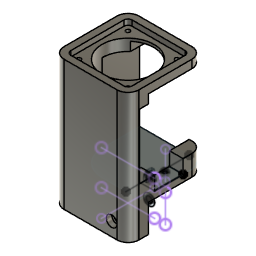
motor-profile connector R (Autodesk Fusion 360 design; units mm, degrees)
Autodesk Fusion 360 part; units mm, degrees
sketch "Sketch1" plane through (0, 0, 0) normal (0, 0, 1) x (1, 0, 0)
  circle A0 centre (0, 0) radius 19
  line L0 (19.5, -22.5) -> (-19.5, -22.5)
  line L1 (-22.5, -19.5) -> (-22.5, 19.5)
  line L2 (-19.5, 22.5) -> (19.5, 22.5)
  line L3 (22.5, 19.5) -> (22.5, -19.5)
  line L4 (22.5, -22.5) -> (-22.5, 22.5) construction
  line L5 (-22.5, -22.5) -> (22.5, 22.5) construction
  line L6 (-2.5, 36.7573) -> (-2.5, -35)
  line L7 (-2.5, -35) -> (-2.5, 36.7573)
  line L8 (-35.201, -2.5) -> (35, -2.5)
  line L9 (35, -2.5) -> (-35.201, -2.5)
  line L10 (7.5, 7.5) -> (62.5, 7.5)
  line L11 (62.5, 7.5) -> (62.5, -12.5)
  line L12 (62.5, -12.5) -> (7.5, -12.5)
  line L13 (7.5, -12.5) -> (7.5, 7.5)
  line L14 (7.5, 7.5) -> (62.5, -12.5) construction
  line L15 (62.5, 7.5) -> (7.5, -12.5) construction
  line L16 (7.5, 7.5) -> (-12.5, 7.5)
  line L17 (-12.5, 7.5) -> (-12.5, 66.0146)
  line L18 (-12.5, 66.0146) -> (7.5, 66.0146)
  line L19 (7.5, 66.0146) -> (7.5, 7.5)
  line L20 (7.5, 7.5) -> (-12.5, 66.0146) construction
  line L21 (-12.5, 7.5) -> (7.5, 66.0146) construction
  circle A1 centre (-18, 18) radius 1.5
  circle A2 centre (18, 18) radius 1.5
  circle A3 centre (-18, -18) radius 1.5
  circle A4 centre (18, -18) radius 1.5
  line L22 (-12.5, 7.5) -> (-12.5, -12.5)
  line L23 (-12.5, -12.5) -> (7.5, -12.5)
  arc A5 (-19.5, 22.5) -> (-22.5, 19.5) centre (-19.5, 19.5) ccw
  arc A6 (-22.5, -19.5) -> (-19.5, -22.5) centre (-19.5, -19.5) ccw
  arc A7 (19.5, -22.5) -> (22.5, -19.5) centre (19.5, -19.5) ccw
  arc A8 (22.5, 19.5) -> (19.5, 22.5) centre (19.5, 19.5) ccw
  arc A9 (-27.5, -19.5) -> (-19.5, -27.5) centre (-19.5, -19.5) ccw
  line L24 (19.5, -27.5) -> (-19.5, -27.5)
  arc A10 (19.5, -27.5) -> (27.5, -19.5) centre (19.5, -19.5) ccw
  line L25 (27.5, 19.5) -> (27.5, -19.5)
  arc A11 (27.5, 19.5) -> (19.5, 27.5) centre (19.5, 19.5) ccw
  line L26 (-19.5, 27.5) -> (19.5, 27.5)
  arc A12 (-19.5, 27.5) -> (-27.5, 19.5) centre (-19.5, 19.5) ccw
  line L27 (-27.5, -19.5) -> (-27.5, 19.5)
  line L28 (-19, 0) -> (-19, 27.5)
  line L29 (0, -19) -> (27.5, -19)
  circle A13 centre (-7, 0) radius 6.5
  point P0 (35, -2.5)
  point P1 (-2.5, 36.7573)
  dimension "d1" = 38
  dimension "d2" = 45
  dimension "d3" = 45
  dimension "d4" = 2.5
  dimension "d5" = 2.5
  dimension "d6" = 20
  dimension "d7" = 4.5
  dimension "d8" = 4.5
  dimension "d9" = 4.5
  dimension "d10" = 4.5
  dimension "d11" = 3
  dimension "d12" = 3
  dimension "d13" = 3
  dimension "d14" = 3
  dimension "d17" = 3
  dimension "d26" = -5
  dimension "d33" = 7
  dimension "d34" = 13
  constraint coincident A0.centre origin
  constraint horizontal L0
  constraint perpendicular L0 L1
  constraint parallel L0 L2
  constraint parallel L1 L3
  constraint coincident L4 A0.centre
  constraint coincident L5 A0.centre
  constraint perpendicular L0 L6
  constraint perpendicular L1 L8
  constraint horizontal L10
  constraint perpendicular L10 L11
  constraint parallel L10 L12
  constraint parallel L11 L13
  constraint coincident L14 P0
  constraint coincident L15 P0
  constraint coincident L5 L10.start
  constraint coincident P0 L8.end
  constraint horizontal L16
  constraint perpendicular L16 L17
  constraint parallel L16 L18
  constraint parallel L17 L19
  constraint coincident L20 P1
  constraint coincident L21 P1
  constraint coincident P1 L6.start
  constraint coincident L4 A1.centre
  constraint coincident L5 A2.centre
  constraint coincident L5 A3.centre
  constraint coincident L4 A4.centre
  constraint coincident L5 L22.end
  constraint perpendicular L16 L22
  constraint coincident L4.end L2
  constraint coincident L4.end L1
  constraint tangent L2 A5
  constraint tangent L1 A5
  constraint coincident L5.start L1
  constraint coincident L5.start L0
  constraint tangent L1 A6
  constraint tangent L0 A6
  constraint equal A5 A6
  constraint coincident L4.start L0
  constraint coincident L4.start L3
  constraint tangent L0 A7
  constraint tangent L3 A7
  constraint equal A5 A7
  constraint coincident L5.end L2
  constraint coincident L5.end L3
  constraint tangent L2 A8
  constraint tangent L3 A8
  constraint equal A5 A8
  constraint coincident A0 L28.start
  constraint coincident L26 L28.end
  constraint perpendicular L26 L28
  constraint coincident A0 L29.start
  constraint coincident L25 L29.end
  constraint perpendicular L25 L29
  measures "d1" diameter of A0
  measures "d2" distance of L4.end L5.end
  measures "d3" distance of L4.start L5.end
  measures "d4" distance of A0.centre L7
  measures "d5" distance of A0.centre L8
  measures "d6" distance of L17.end L18.end
  measures "d7" distance of L2 A1.centre
  measures "d8" distance of L2 A2.centre
  measures "d9" distance of L0 A3.centre
  measures "d10" distance of L0 A4.centre
  measures "d11" diameter of A1
  measures "d12" diameter of A2
  measures "d13" diameter of A4
  measures "d14" diameter of A3
  measures "d17" radius of A5
  measures "d33" distance of A0.centre A13.centre
  measures "d34" diameter of A13
extrude "Extrude1" add sketch "Sketch1" along normal blind 95.5 contours A0 L3 L12 A4 L29 | A0 L6 L7 L12 L23 | A0 L0 L3 L6 L7 A4 A7 L29 | L3 L12 L25 L29 | A0 L8 L9 L17 L22 A13 | A0 L2 L17 A1 L28 | A0 L0 L1 L6 L7 L8 L9 A6 | A0 L6 L7 L8 L9 L22 L23 A13 | A4 L29 | A4 L29 | L0 L3 L6 L7 A7 L24 A10 L25 L29 | A0 L1 L2 L8 L9 A1 A5 L28 | L2 L17 L26 L28 | L8 L9 L22 A13 | L0 L1 L6 L7 L8 L9 A6 A9 L24 L27 | L8 L9 L22 A13 | A1 L28 | A1 L28 | L1 L2 L8 L9 A5 L26 A12 L27 L28 | A3
extrude "Extrude2" add sketch "Sketch1" along normal blind 6 from surface at 89.5 contours A0 L3 L8 L9 L10 | A0 L2 L3 L10 L19 A8 | A0 L3 L8 L9 L12 | A0 L2 L6 L7 L19 | L3 L8 L9 L10 L25 | L2 L3 L10 L19 A8 L25 A11 L26 | A0 L3 L12 A4 L29 | L3 L8 L9 L12 L25 | A0 L2 L6 L7 L17 | L2 L6 L7 L19 L26 | A0 L0 L3 L6 L7 A4 A7 L29 | L3 L12 L25 L29 | A0 L2 L17 A1 L28 | L2 L6 L7 L17 L26 | A0 L0 L1 L6 L7 L8 L9 A6 | A4 L29 | A4 L29 | L0 L3 L6 L7 A7 L24 A10 L25 L29 | A0 L1 L2 L8 L9 A1 A5 L28 | L2 L17 L26 L28 | L0 L1 L6 L7 L8 L9 A6 A9 L24 L27 | A1 L28 | A1 L28 | L1 L2 L8 L9 A5 L26 A12 L27 L28 | A2 | A3
extrude "Extrude5" cut sketch "Sketch1" along normal blind 4 from surface at 91.5 contours A0 L8 L9 L10 L13 | A0 L3 L8 L9 L10 | A0 L10 L19 | A0 L2 L3 L10 L19 A8 | A0 L3 L8 L9 L12 | A0 L8 L9 L12 L13 | A0 L6 L7 L16 L19 | A0 L2 L6 L7 L19 | L6 L7 L8 L9 L13 L16 A13 | A0 L3 L12 A4 L29 | A0 L6 L7 L12 L23 | L6 L7 L8 L9 L13 L23 A13 | A0 L6 L7 L16 L17 | A0 L2 L6 L7 L17 | L6 L7 L16 L22 A13 | A0 L0 L3 L6 L7 A4 A7 L29 | L6 L7 L8 L9 A13 | L6 L7 L8 L9 A13 | A0 L8 L9 L17 L22 A13 | A0 L2 L17 A1 L28 | L6 L7 L8 L9 L22 A13 | A0 L0 L1 L6 L7 L8 L9 A6 | A0 L6 L7 L8 L9 L22 L23 A13 | A4 L29 | A4 L29 | L6 L7 L22 L23 A13 | L6 L7 L8 L9 L22 A13 | A0 L1 L2 L8 L9 A1 A5 L28 | L8 L9 L22 A13 | L8 L9 L22 A13 | A1 L28 | A1 L28 | A2 | A3
extrude "Extrude3" cut sketch "Sketch1" along normal blind 8 from surface at 83.5 contours A4 L29 | A4 L29 | A1 L28 | A1 L28 | A2 | A3
extrude "Extrude4" cut sketch "Sketch1" along normal through all from surface at 20.5 contours A0 L8 L9 L10 L13 | A0 L10 L19 | A0 L8 L9 L12 L13 | A0 L6 L7 L16 L19 | L6 L7 L8 L9 L13 L16 A13 | A0 L6 L7 L12 L23 | L6 L7 L8 L9 L13 L23 A13 | A0 L6 L7 L16 L17 | L6 L7 L16 L22 A13 | L6 L7 L8 L9 A13 | L6 L7 L8 L9 A13 | A0 L8 L9 L17 L22 A13 | L6 L7 L8 L9 L22 A13 | A0 L6 L7 L8 L9 L22 L23 A13 | L6 L7 L22 L23 A13 | L6 L7 L8 L9 L22 A13 | L8 L9 L22 A13 | L8 L9 L22 A13
extrude "Extrude6" cut sketch "Sketch1" along normal blind 62.5 from surface at 20.5 contours A0 L3 L12 A4 L29 | L3 L12 L25 L29 | A0 L2 L17 A1 L28 | A4 L29 | L2 L17 L26 L28 | A1 L28 picked at (17.9212, -18.1088) picked at (-18.2904, 18.3293)
extrude "Extrude7" add sketch "Sketch1" 1 faces at (-17.5, 11.5, 0) along normal blind 5 from surface at 20.5 contours A0 L8 L9 L10 L13 | A0 L3 L8 L9 L10 | A0 L10 L19 | A0 L2 L3 L10 L19 A8 | A0 L3 L8 L9 L12 | A0 L8 L9 L12 L13 | A0 L6 L7 L16 L19 | A0 L2 L6 L7 L19 | L6 L7 L8 L9 L13 L16 A13 | L3 L8 L9 L10 L25 | L2 L3 L10 L19 A8 L25 A11 L26 | A0 L3 L12 A4 L29 | A0 L6 L7 L12 L23 | L6 L7 L8 L9 L13 L23 A13 | L3 L8 L9 L12 L25 | A0 L6 L7 L16 L17 | A0 L2 L6 L7 L17 | L2 L6 L7 L19 L26 | L6 L7 L16 L22 A13 | L3 L12 L25 L29 | L6 L7 L8 L9 A13 | L6 L7 L8 L9 A13 | A0 L8 L9 L17 L22 A13 | A0 L2 L17 A1 L28 | L2 L6 L7 L17 L26 | L6 L7 L8 L9 L22 A13 | A0 L0 L1 L6 L7 L8 L9 A6 | A0 L6 L7 L8 L9 L22 L23 A13 | L6 L7 L22 L23 A13 | L6 L7 L8 L9 L22 A13 | A0 L1 L2 L8 L9 A1 A5 L28 | L2 L17 L26 L28 | L8 L9 L22 A13 | L0 L1 L6 L7 L8 L9 A6 A9 L24 L27 | L8 L9 L22 A13 | A1 L28 | A1 L28 | L1 L2 L8 L9 A5 L26 A12 L27 L28 | A2 | A3
sketch "Sketch2" plane through (0, 0, 0) normal (1, 0, 0) x (0, 1, 0)
  circle A0 centre (15.5, 10) radius 2.1
  circle A1 centre (15.5, 10) radius 4
  line L0 (19.5, 0) -> (-19.5, 0)
  line L1 (27.5, 0) -> (27.5, 20.5)
  line L2 (17.5, 13.4641) -> (17.5, 6.5359)
  line L3 (13.5, 13.4641) -> (13.5, 6.5359)
  line L4 (12.0359, 12) -> (18.9641, 12)
  line L5 (12.0359, 8) -> (18.9641, 8)
  dimension "d38" = 10
  dimension "d39" = 4.2
  dimension "d40" = 8
  dimension "d41" = 12
  dimension "d54" = 2
  dimension "d55" = 2
  dimension "d56" = 2
  dimension "d57" = 2
  constraint concentric A0 A1
  constraint coincident A1 L2.start
  constraint coincident A1 L2.end
  constraint vertical L2
  constraint coincident A1 L3.start
  constraint coincident A1 L3.end
  constraint parallel L2 L3
  constraint coincident A1 L4.start
  constraint coincident A1 L4.end
  constraint perpendicular L3 L4
  constraint coincident A1 L5.start
  constraint coincident A1 L5.end
  constraint perpendicular L3 L5
  measures "d38" distance of A0.centre L0
  measures "d39" diameter of A0
  measures "d40" diameter of A1
  measures "d41" distance of A0.centre L1
  measures "d54" distance of A0.centre L3
  measures "d55" distance of A0.centre L2
  measures "d56" distance of A0.centre L4
  measures "d57" distance of A0.centre L5
extrude "Extrude8" cut sketch "Sketch2" against normal through all contours A0 L2 | A0 L2 L3 L4 L5 | A0 L4 | A0 L5 | A0 L3
extrude "Extrude9" cut sketch "Sketch2" against normal blind 4 from surface at -23.5 contours A0 A1 L2 L4 L5 | A0 L2 L4 | A0 L2 L5 | A0 A1 L2 L3 L4 | A1 L2 L4 | A0 A1 L2 L3 L5 | A1 L2 L5 | A0 L3 L4 | A0 L3 L5 | A0 A1 L3 L4 L5 | A1 L3 L4 | A1 L3 L5
sketch "Sketch3" plane through (0, 0, 0) normal (0, 1, 0) x (1, 0, 0)
  circle A0 centre (15.5, -10) radius 2.1
  circle A1 centre (15.5, -10) radius 4
  line L0 (-19.5, 0) -> (19.5, 0)
  line L1 (27.5, 0) -> (27.5, -20.5)
  dimension "d46" = 10
  dimension "d47" = 4.2
  dimension "d48" = 8
  dimension "d49" = 12
  constraint concentric A0 A1
  measures "d46" distance of A0.centre L0
  measures "d47" diameter of A0
  measures "d48" diameter of A1
  measures "d49" distance of A0.centre L1
extrude "Extrude10" cut sketch "Sketch3" against normal through all contours A0
extrude "Extrude11" cut sketch "Sketch3" along normal blind 4 from surface at -27.5
extrude "Extrude12" add sketch "Sketch2" against normal blind 0.2 from surface at -23.5 contours A0 L2 | A0 A1 L2 L4 L5 | A1 L2 L4 | A1 L2 L5 | A0 L3 | A0 A1 L3 L4 L5 | A1 L3 L4 | A1 L3 L5
extrude "Extrude13" add sketch "Sketch2" against normal blind 0.4 from surface at -23.5 contours A0 L4 | A0 A1 L2 L3 L4 | A1 L2 L4 | A0 A1 L2 L3 L5 | A0 L5 | A1 L2 L5 | A1 L3 L4 | A1 L3 L5
sketch "Sketch5" plane through (0, 0, 25.5) normal (0, 0, 1) x (-1, 0, 0)
  line L0 (19, -27.5) -> (19, 0)
  arc A0 (19, 0) -> (0, 19) centre (0, 0) ccw
  line L1 (0, 19) -> (-27.5, 19)
  line L2 (-27.5, 19) -> (-27.5, -19.5)
  arc A1 (-27.5, -19.5) -> (-19.5, -27.5) centre (-19.5, -19.5) ccw
  line L3 (-19.5, -27.5) -> (19, -27.5)
  line L4 (-27.5, -13) -> (-17.5, -13)
  line L5 (-17.5, -13) -> (-17.5, 8)
  line L6 (-17.5, 8) -> (-27.5, 8)
  line L7 (-27.5, 8) -> (-27.5, -13)
  line L8 (19.5, 0) -> (-19.5, 0)
  circle A2 centre (-19.5, -7.5) radius 1.05
  circle A3 centre (-19.5, 2.5) radius 1.05
  line L9 (-17.5, 8) -> (-17.5, 19)
  line L10 (-17.5, -13) -> (-17.5, -27.5)
  dimension "d64" = 21
  dimension "d65" = 13
  dimension "d66" = 10
  dimension "d67" = 2.1
  dimension "d68" = 2.1
  dimension "d69" = 5.5
  dimension "d70" = 5.5
  dimension "d71" = 8
  dimension "d72" = 8
  constraint horizontal L4
  constraint vertical L5
  constraint horizontal L6
  constraint vertical L7
  constraint coincident L2 L4.start
  constraint coincident L1 L9.end
  constraint perpendicular L1 L9
  constraint coincident L3 L10.end
  constraint perpendicular L3 L10
  measures "d64" distance of L4.start L6.end
  measures "d65" distance of L4 L8
  measures "d66" distance of L5.end L6.end
  measures "d67" diameter of A2
  measures "d68" diameter of A3
  measures "d69" distance of L4 A2.centre
  measures "d70" distance of L6 A3.centre
  measures "d71" distance of L7 A3.centre
  measures "d72" distance of L7 A2.centre
extrude "Extrude14" add sketch "Sketch5" along normal blind 10 contours L2 A1 L3 L4 L10 | L1 L2 L6 L9
extrude "Extrude15" cut sketch "Sketch5" against normal through all contours A2 | A3
